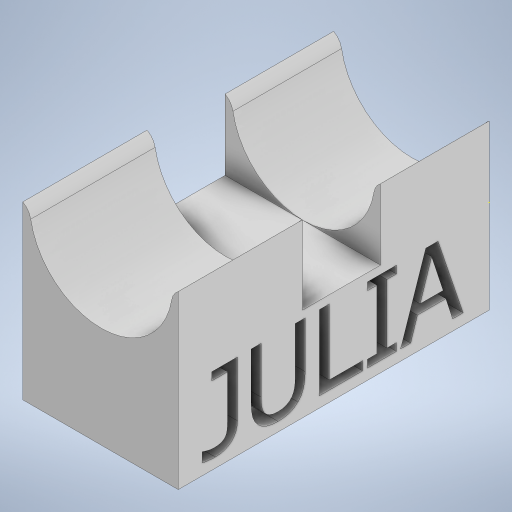
# Autodesk Inventor part: MAKO
Saved by Autodesk Inventor 2023 (Build 270158000, 158)
## iProperties
Created: 2022-12-21
Part Number: MAKO
Material: Generic
Document SubType Name: Modeling
Designer: julia
Density: 1 g/cm^3
Appearance: Default
Author: julia
Autodesk Inventor part; units mm, degrees
ref_plane "YZ Plane" through (0, 0, 0) normal (1, 0, 0) x (0, 1, 0)
ref_plane "XZ Plane" through (0, 0, 0) normal (0, 1, 0) x (-1, 0, 0)
ref_plane "XY Plane" through (0, 0, 0) normal (0, 0, 1) x (1, 0, 0)
sketch "Sketch1" plane through (0, 0, 0) normal (0, 1, 0) x (-1, 0, 0)
  line L0 (0, 0) -> (2.5, 0)
  line L1 (2.5, 0) -> (2.5, 5)
  line L2 (2.5, 5) -> (0, 5)
  line L3 (0, 5) -> (0, 0)
  dimension "d0" = 2.5
  dimension "d1" = 5
  constraints: 8 end point, 2 parallel, 1 horizontal, 1 perpendicular
  measures "d0" distance of L2.end L1.end
  measures "d1" distance of L1.end L0.end
extrude "Extrusion1" add sketch "Sketch1" along normal blind 1.5
sketch "Sketch2" plane through (0, 1.5, 0) normal (0, 1, 0) x (1, 0, 0)
  line L0 (0, -5) -> (0, 0) projected
  line L1 (-2.5, 0) -> (-2.5, -5) projected
  line L2 (0, -5) -> (-2.5, -5)
  line L3 (-2.5, -5) -> (-2.5, -3)
  line L4 (-2.5, -3) -> (0, -3)
  line L5 (0, -3) -> (0, -5)
  dimension "d4" = 2
  constraints: 8 end point, 2 parallel, 1 horizontal, 1 perpendicular, 1 point on line
  measures "d4" distance of L2.end L3.end
extrude "Extrusion2" add sketch "Sketch2" along normal blind 2.6
sketch "Sketch3" plane through (0, 1.5, 3) normal (0, 0, -1) x (-1, 0, 0)
  circle A0 centre (1.2397, 1.278) radius 1.15
  point P0 (0, -1.5)
  dimension "d7" = 2.3
  constraints: 1 centre point
  measures "d7" diameter of A0
extrude "Extrusion3" cut sketch "Sketch3" against normal blind 3.75
fillet "Fillet1" radius 0.25 1 edges at (0, 4.1, 4)
fillet "Fillet2" radius 0.25 1 edges at (-2.5, 4.1, 4)
sketch "Sketch4" plane through (0, 1.5, 3) normal (0, 0, -1) x (-1, 0, 0)
  line L0 (0, -1.5) -> (0, 2.35) projected
  line L1 (0, 1.2577) -> (2.5, 1.2577)
  line L2 (2.5, 1.2577) -> (2.5, 2.6)
  line L3 (2.5, 2.6) -> (0, 2.6)
  line L4 (0, 2.6) -> (0, 1.2577)
  constraints: 8 end point, 2 parallel, 1 horizontal, 1 perpendicular, 1 point on line
extrude "Extrusion4" cut sketch "Sketch4" against normal blind 3.75
fillet "Fillet3" radius 0.25 2 edges at (-0.0899, 2.7577, 4) (-2.3895, 2.7577, 4)
fillet_without_effect "Fillet4"
sketch "Sketch5" plane through (0, 1.5, 0) normal (0, 1, 0) x (1, 0, 0)
  point P0 (0, 0)
sketch "Sketch6" plane through (0, 0, 5) normal (1, 0, 0) x (0, 0, -1)
  line L0 (-0.0284, 1.4498) -> (4.996, 1.4498) construction
  line L1 (4.996, 1.4498) -> (4.996, 0.0679) construction
  line L2 (4.996, 0.0679) -> (-0.0284, 0.0679) construction
  line L3 (-0.0284, 0.0679) -> (-0.0284, 1.4498) construction
  spline S0 degree 2 poles (0.9517, 0.4837) (0.9517, 0.3261) (0.7592, 0.155) (0.5968, 0.155) knots 0 0 0 1 2 2 2
  spline S1 degree 2 poles (0.5968, 0.155) (0.5579, 0.155) (0.4285, 0.1686) (0.3848, 0.1783) knots 0 0 0 1 2 2 2
  line L4 (0.3848, 0.1783) -> (0.3848, 0.332)
  line L5 (0.3848, 0.332) -> (0.3935, 0.332)
  spline S2 degree 2 poles (0.3935, 0.332) (0.4266, 0.3203) (0.5248, 0.2931) (0.5754, 0.2931) knots 0 0 0 1 2 2 2
  spline S3 degree 2 poles (0.5754, 0.2931) (0.6493, 0.2931) (0.7378, 0.3271) (0.7582, 0.3582) knots 0 0 0 1 2 2 2
  spline S4 degree 2 poles (0.7582, 0.3582) (0.7805, 0.3903) (0.7922, 0.4837) (0.7922, 0.5449) knots 0 0 0 1 2 2 2
  line L6 (0.7922, 0.5449) -> (0.7922, 1.2441)
  line L7 (0.7922, 1.2441) -> (0.5384, 1.2441)
  line L8 (0.5384, 1.2441) -> (0.5384, 1.3715)
  line L9 (0.5384, 1.3715) -> (0.9517, 1.3715)
  line L10 (0.9517, 1.3715) -> (0.9517, 0.4837)
  spline S5 degree 2 poles (1.6062, 0.1462) (1.5002, 0.1462) (1.3426, 0.2016) (1.2872, 0.2571) knots 0 0 0 1 2 2 2
  spline S6 degree 2 poles (1.2872, 0.2571) (1.224, 0.3193) (1.1724, 0.4944) (1.1724, 0.6227) knots 0 0 0 1 2 2 2
  line L11 (1.1724, 0.6227) -> (1.1724, 1.3715)
  line L12 (1.1724, 1.3715) -> (1.3319, 1.3715)
  line L13 (1.3319, 1.3715) -> (1.3319, 0.6227)
  spline S7 degree 2 poles (1.3319, 0.6227) (1.3319, 0.5391) (1.3533, 0.4263) (1.3835, 0.3806) knots 0 0 0 1 2 2 2
  spline S8 degree 2 poles (1.3835, 0.3806) (1.4156, 0.332) (1.5264, 0.2824) (1.6062, 0.2824) knots 0 0 0 1 2 2 2
  spline S9 degree 2 poles (1.6062, 0.2824) (1.681, 0.2824) (1.7977, 0.332) (1.8298, 0.3806) knots 0 0 0 1 2 2 2
  spline S10 degree 2 poles (1.8298, 0.3806) (1.86, 0.4263) (1.8814, 0.5381) (1.8814, 0.6188) knots 0 0 0 1 2 2 2
  line L14 (1.8814, 0.6188) -> (1.8814, 1.3715)
  line L15 (1.8814, 1.3715) -> (2.0408, 1.3715)
  line L16 (2.0408, 1.3715) -> (2.0408, 0.6227)
  spline S11 degree 2 poles (2.0408, 0.6227) (2.0408, 0.4973) (1.9903, 0.3183) (1.9261, 0.2571) knots 0 0 0 1 2 2 2
  spline S12 degree 2 poles (1.9261, 0.2571) (1.8687, 0.2007) (1.717, 0.1462) (1.6062, 0.1462) knots 0 0 0 1 2 2 2
  line L17 (2.9647, 0.1715) -> (2.2694, 0.1715)
  line L18 (2.2694, 0.1715) -> (2.2694, 1.3715)
  line L19 (2.2694, 1.3715) -> (2.4288, 1.3715)
  line L20 (2.4288, 1.3715) -> (2.4288, 0.3135)
  line L21 (2.4288, 0.3135) -> (2.9647, 0.3135)
  line L22 (2.9647, 0.3135) -> (2.9647, 0.1715)
  line L23 (3.5083, 0.1715) -> (3.0434, 0.1715)
  line L24 (3.0434, 0.1715) -> (3.0434, 0.294)
  line L25 (3.0434, 0.294) -> (3.1961, 0.294)
  line L26 (3.1961, 0.294) -> (3.1961, 1.249)
  line L27 (3.1961, 1.249) -> (3.0434, 1.249)
  line L28 (3.0434, 1.249) -> (3.0434, 1.3715)
  line L29 (3.0434, 1.3715) -> (3.5083, 1.3715)
  line L30 (3.5083, 1.3715) -> (3.5083, 1.249)
  line L31 (3.5083, 1.249) -> (3.3556, 1.249)
  line L32 (3.3556, 1.249) -> (3.3556, 0.294)
  line L33 (3.3556, 0.294) -> (3.5083, 0.294)
  line L34 (3.5083, 0.294) -> (3.5083, 0.1715)
  line L35 (3.5763, 0.1715) -> (3.9809, 1.3715)
  line L36 (3.9809, 1.3715) -> (4.1773, 1.3715)
  line L37 (4.1773, 1.3715) -> (4.5818, 0.1715)
  line L38 (4.5818, 0.1715) -> (4.4136, 0.1715)
  line L39 (4.4136, 0.1715) -> (4.3047, 0.507)
  line L40 (4.3047, 0.507) -> (3.8467, 0.507)
  line L41 (3.8467, 0.507) -> (3.7378, 0.1715)
  line L42 (3.7378, 0.1715) -> (3.5763, 0.1715)
  line L43 (4.2609, 0.6431) -> (4.0752, 1.2081)
  line L44 (4.0752, 1.2081) -> (3.8904, 0.6431)
  line L45 (3.8904, 0.6431) -> (4.2609, 0.6431)
  point P0 (5, 0)
  constraints: 2 other
emboss "Emboss1" sketch "Sketch6" operation cut depth 0.5 direction (-1, 0, 0)
sketch "Sketch7" plane through (-2.5, 0, 0) normal (-1, 0, 0) x (0, 0, 1)
  line L0 (0.0799, 1.3842) -> (4.9393, 1.3842) construction
  line L1 (4.9393, 1.3842) -> (4.9393, 0.1336) construction
  line L2 (4.9393, 0.1336) -> (0.0799, 0.1336) construction
  line L3 (0.0799, 0.1336) -> (0.0799, 1.3842) construction
  spline S0 degree 2 poles (0.96, 0.9972) (0.96, 0.9194) (0.9046, 0.7793) (0.855, 0.7307) knots 0 0 0 1 2 2 2
  spline S1 degree 2 poles (0.855, 0.7307) (0.7927, 0.6694) (0.6245, 0.6062) (0.4961, 0.6062) knots 0 0 0 1 2 2 2
  line L4 (0.4961, 0.6062) -> (0.361, 0.6062)
  line L5 (0.361, 0.6062) -> (0.361, 0.1589)
  line L6 (0.361, 0.1589) -> (0.2015, 0.1589)
  line L7 (0.2015, 0.1589) -> (0.2015, 1.3589)
  line L8 (0.2015, 1.3589) -> (0.5029, 1.3589)
  spline S2 degree 2 poles (0.5029, 1.3589) (0.6099, 1.3589) (0.7597, 1.3239) (0.817, 1.284) knots 0 0 0 1 2 2 2
  spline S3 degree 2 poles (0.817, 1.284) (0.8841, 1.2383) (0.96, 1.0973) (0.96, 0.9972) knots 0 0 0 1 2 2 2
  spline S4 degree 2 poles (0.7937, 0.9923) (0.7937, 1.0545) (0.7509, 1.1459) (0.7072, 1.1751) knots 0 0 0 1 2 2 2
  spline S5 degree 2 poles (0.7072, 1.1751) (0.6692, 1.2004) (0.5681, 1.2208) (0.4932, 1.2208) knots 0 0 0 1 2 2 2
  line L9 (0.4932, 1.2208) -> (0.361, 1.2208)
  line L10 (0.361, 1.2208) -> (0.361, 0.7424)
  line L11 (0.361, 0.7424) -> (0.4699, 0.7424)
  spline S6 degree 2 poles (0.4699, 0.7424) (0.5671, 0.7424) (0.6867, 0.7735) (0.7256, 0.8143) knots 0 0 0 1 2 2 2
  spline S7 degree 2 poles (0.7256, 0.8143) (0.7616, 0.8503) (0.7937, 0.9349) (0.7937, 0.9923) knots 0 0 0 1 2 2 2
  spline S8 degree 2 poles (1.9606, 1.2218) (2.0287, 1.142) (2.1046, 0.9087) (2.1046, 0.7589) knots 0 0 0 1 2 2 2
  spline S9 degree 2 poles (2.1046, 0.7589) (2.1046, 0.613) (2.0307, 0.3767) (1.9606, 0.297) knots 0 0 0 1 2 2 2
  spline S10 degree 2 poles (1.9606, 0.297) (1.8867, 0.2134) (1.6913, 0.1336) (1.5736, 0.1336) knots 0 0 0 1 2 2 2
  spline S11 degree 2 poles (1.5736, 0.1336) (1.4521, 0.1336) (1.2576, 0.2163) (1.1866, 0.297) knots 0 0 0 1 2 2 2
  spline S12 degree 2 poles (1.1866, 0.297) (1.1175, 0.3767) (1.0436, 0.6111) (1.0436, 0.7589) knots 0 0 0 1 2 2 2
  spline S13 degree 2 poles (1.0436, 0.7589) (1.0436, 0.9096) (1.1185, 1.1391) (1.1876, 1.2218) knots 0 0 0 1 2 2 2
  spline S14 degree 2 poles (1.1876, 1.2218) (1.2576, 1.3015) (1.453, 1.3842) (1.5736, 1.3842) knots 0 0 0 1 2 2 2
  spline S15 degree 2 poles (1.5736, 1.3842) (1.6961, 1.3842) (1.8926, 1.2986) (1.9606, 1.2218) knots 0 0 0 1 2 2 2
  spline S16 degree 2 poles (1.9383, 0.7589) (1.9383, 0.8775) (1.8867, 1.0613) (1.8401, 1.1216) knots 0 0 0 1 2 2 2
  spline S17 degree 2 poles (1.8401, 1.1216) (1.7924, 1.1839) (1.6582, 1.2461) (1.5746, 1.2461) knots 0 0 0 1 2 2 2
  spline S18 degree 2 poles (1.5746, 1.2461) (1.488, 1.2461) (1.3577, 1.1858) (1.3081, 1.1216) knots 0 0 0 1 2 2 2
  spline S19 degree 2 poles (1.3081, 1.1216) (1.2605, 1.0604) (1.2099, 0.8756) (1.2099, 0.7589) knots 0 0 0 1 2 2 2
  spline S20 degree 2 poles (1.2099, 0.7589) (1.2099, 0.5226) (1.4083, 0.2717) (1.5746, 0.2717) knots 0 0 0 1 2 2 2
  spline S21 degree 2 poles (1.5746, 0.2717) (1.7409, 0.2717) (1.9383, 0.5226) (1.9383, 0.7589) knots 0 0 0 1 2 2 2
  line L12 (2.9749, 0.1589) -> (2.2796, 0.1589)
  line L13 (2.2796, 0.1589) -> (2.2796, 1.3589)
  line L14 (2.2796, 1.3589) -> (2.4391, 1.3589)
  line L15 (2.4391, 1.3589) -> (2.4391, 0.3009)
  line L16 (2.4391, 0.3009) -> (2.9749, 0.3009)
  line L17 (2.9749, 0.3009) -> (2.9749, 0.1589)
  line L18 (2.971, 0.1589) -> (3.3756, 1.3589)
  line L19 (3.3756, 1.3589) -> (3.572, 1.3589)
  line L20 (3.572, 1.3589) -> (3.9765, 0.1589)
  line L21 (3.9765, 0.1589) -> (3.8083, 0.1589)
  line L22 (3.8083, 0.1589) -> (3.6994, 0.4944)
  line L23 (3.6994, 0.4944) -> (3.2414, 0.4944)
  line L24 (3.2414, 0.4944) -> (3.1324, 0.1589)
  line L25 (3.1324, 0.1589) -> (2.971, 0.1589)
  line L26 (3.6556, 0.6305) -> (3.4699, 1.1955)
  line L27 (3.4699, 1.1955) -> (3.2851, 0.6305)
  line L28 (3.2851, 0.6305) -> (3.6556, 0.6305)
  line L29 (4.9655, 0.1589) -> (4.7584, 0.1589)
  line L30 (4.7584, 0.1589) -> (4.3198, 0.7171)
  line L31 (4.3198, 0.7171) -> (4.2498, 0.6383)
  line L32 (4.2498, 0.6383) -> (4.2498, 0.1589)
  line L33 (4.2498, 0.1589) -> (4.0903, 0.1589)
  line L34 (4.0903, 0.1589) -> (4.0903, 1.3589)
  line L35 (4.0903, 1.3589) -> (4.2498, 1.3589)
  line L36 (4.2498, 1.3589) -> (4.2498, 0.8075)
  line L37 (4.2498, 0.8075) -> (4.7418, 1.3589)
  line L38 (4.7418, 1.3589) -> (4.9363, 1.3589)
  line L39 (4.9363, 1.3589) -> (4.4394, 0.8231)
  line L40 (4.4394, 0.8231) -> (4.9655, 0.1589)
  point P0 (0, 0)
  constraints: 2 other
emboss "Emboss2" sketch "Sketch7" operation cut depth 0.5 direction (1, 0, 0)
sketch "Sketch8" plane through (0, 1.5, 0) normal (0, 1, 0) x (1, 0, 0)
  line L0 (-2.5, 0) -> (-2.5, -5) projected
  line L1 (0, -5) -> (0, 0) projected
  line L2 (-2.5, -1.7467) -> (0, -1.7467)
  line L3 (0, -1.7467) -> (0, 0)
  line L4 (0, 0) -> (-2.5, 0)
  line L5 (-2.5, 0) -> (-2.5, -1.7467)
  constraints: 8 end point, 2 parallel, 1 horizontal, 1 perpendicular, 1 point on line
extrude "Extrusion5" add sketch "Sketch8" along normal blind 2.5
sketch "Sketch9" plane through (-2.5, 1.5, 1.7467) normal (0, 0, 1) x (1, 0, 0)
  circle A0 centre (1.2603, 1.1506) radius 1.15
  point P0 (2.5, -1.5)
  dimension "d22" = 2.3
  constraints: 1 centre point
  measures "d22" diameter of A0
extrude "Extrusion6" cut sketch "Sketch9" against normal blind 2
sketch "Sketch10" plane through (0, 0, 0) normal (0, 0, -1) x (-1, 0, 0)
  line L0 (0, 1.5) -> (0, 4) projected
  line L1 (2.5, 1.5) -> (2.5, 4) projected
  line L2 (0, 4) -> (2.5, 4)
  line L3 (2.5, 4) -> (2.5, 2.6337)
  line L4 (2.5, 2.6337) -> (0, 2.6337)
  line L5 (0, 2.6337) -> (0, 4)
  point P0 (0, 0)
  constraints: 8 end point, 2 parallel, 1 horizontal, 1 perpendicular, 1 point on line
extrude "Extrusion7" cut sketch "Sketch10" against normal blind 2
fillet "Fillet5" radius 0.25 2 edges at (-2.3896, 2.6337, 0.8733) (-0.0898, 2.6337, 0.8733)
fillet_without_effect "Fillet6"
body "Solid1"
